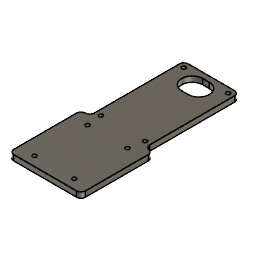
LiDAR MOUNT (Autodesk Fusion 360 design; units mm, degrees)
Autodesk Fusion 360 part; units mm, degrees
note: some values were not read from the file. Set by a fixed rule: the direction of a hole.
sketch "Sketch1" plane through (0, 0, 0) normal (0, 0, 1) x (1, 0, 0)
  line L0 (-32.5, 32.5) -> (32.5, 32.5)
  line L1 (32.5, 32.5) -> (32.5, -32.5)
  line L2 (32.5, -32.5) -> (-32.5, -32.5)
  line L3 (-32.5, -32.5) -> (-32.5, 32.5)
  point P0 (-18, 24)
  point P1 (18, 24)
  point P2 (18, -24)
  point P3 (-18, -24)
  dimension "d1" = 65
  dimension "d2" = 65
  dimension "d3" = 32.5
  dimension "d4" = 32.5
  dimension "d5" = 14.5
  dimension "d6" = 14.5
  dimension "d7" = 14.5
  dimension "d8" = 14.5
  dimension "d9" = 8.5
  dimension "d10" = 8.5
  dimension "d11" = 8.5
  dimension "d12" = 8.5
  constraint horizontal L0
  constraint vertical L1
  constraint horizontal L2
  constraint vertical L3
  measures "d1" distance of L0.start L2.end
  measures "d2" distance of L0.start L0.end
  measures "d3" distance of origin L3
  measures "d4" distance of origin L2
  measures "d5" distance of L1 P2
  measures "d6" distance of L1 P1
  measures "d7" distance of L3 P0
  measures "d8" distance of L3 P3
  measures "d9" distance of L2 P3
  measures "d10" distance of L0 P0
  measures "d11" distance of L0 P1
  measures "d12" distance of L2 P2
extrude "Extrude1" add sketch "Sketch1" along normal blind 5
hole "Hole1" at (-18, -24, 0) at (18, -24, 0) at (18, 24, 0) at (-18, 24, 0) direction (0, 0, 1) diameter 3.5 depth 5 tip angle 180 countersink diameter 6 countersink angle 90
sketch "Sketch2" plane through (0, 32.5, 0) normal (0, 1, 0) x (-1, 0, 0)
  line L0 (-32.5, 0) -> (32.5, 0)
  line L1 (32.5, 0) -> (32.5, 5)
  line L2 (32.5, 5) -> (-32.5, 5)
  line L3 (-32.5, 5) -> (-32.5, 0)
  line L4 (-25.5, 5) -> (24.5, 5)
  line L5 (24.5, 5) -> (24.5, 0)
  line L6 (24.5, 0) -> (-25.5, 0)
  line L7 (-25.5, 0) -> (-25.5, 5)
  dimension "d20" = 50
  dimension "d21" = 7
  constraint horizontal L4
  constraint vertical L5
  constraint horizontal L6
  constraint vertical L7
  constraint coincident L2 L4.start
  measures "d20" distance of L4.start L4.end
  measures "d21" distance of L3 L7
extrude "Extrude2" add sketch "Sketch2" along normal blind 85 contours L0 L2 L4 L5 L6 L7
sketch "Sketch3" plane through (0, 0, 5) normal (0, 0, 1) x (-1, 0, 0)
  circle A0 centre (-18, -24) radius 1.75
  circle A1 centre (18, 24) radius 1.75
  circle A2 centre (-18, 24) radius 1.75
  circle A3 centre (18, -24) radius 1.75
  line L0 (32.5, 32.5) -> (-32.5, 32.5)
  line L1 (-32.5, 32.5) -> (-32.5, -32.5)
  line L2 (-32.5, -32.5) -> (-25.5, -32.5)
  line L3 (-25.5, -32.5) -> (-25.5, -117.5)
  line L4 (-25.5, -117.5) -> (24.5, -117.5)
  line L5 (24.5, -117.5) -> (24.5, -32.5)
  line L6 (24.5, -32.5) -> (32.5, -32.5)
  line L7 (32.5, -32.5) -> (32.5, 32.5)
  line L8 (24.5, -32.5) -> (-25.5, -32.5) construction
  line L9 (2.5, -112.5) -> (-3.5, -112.5)
  line L10 (2.5, -93.5) -> (-3.5, -93.5)
  arc A4 (-3.5, -93.5) -> (-3.5, -112.5) centre (-3.5, -103) ccw
  arc A5 (2.5, -112.5) -> (2.5, -93.5) centre (2.5, -103) ccw
  circle A6 centre (19.5, -37.5) radius 1.75
  circle A7 centre (-20.5, -37.5) radius 1.75
  circle A8 centre (-20.5, -112.5) radius 1.75
  circle A9 centre (19.5, -112.5) radius 1.75
  point P0 (12, -103)
  point P1 (-13, -103)
  dimension "d27" = 19
  dimension "d29" = 22
  dimension "d30" = 3.5
  dimension "d31" = 3.5
  dimension "d32" = 3.5
  dimension "d33" = 3.5
  dimension "d34" = 5
  dimension "d35" = 5
  dimension "d36" = 5
  dimension "d37" = 5
  dimension "d39" = 5
  dimension "d40" = 5
  dimension "d48" = 22
  dimension "d49" = 5
  constraint coincident L5.end L6.start
  constraint coincident L2.end L3.start
  constraint tangent L9 A4
  constraint tangent L9 A5
  constraint tangent L10 A4
  constraint tangent L10 A5
  constraint horizontal A5.centre A4.centre
  constraint midpoint A5 P0
  constraint midpoint A4 P1
  measures "d27" distance of L9 L10
  measures "d29" distance of L5 A5.centre
  measures "d30" diameter of A6
  measures "d31" diameter of A7
  measures "d32" diameter of A8
  measures "d33" diameter of A9
  measures "d34" distance of L8 A6.centre
  measures "d35" distance of L5 A6.centre
  measures "d36" distance of L3 A7.centre
  measures "d37" distance of L8 A7.centre
  measures "d39" distance of L5 A9.centre
  measures "d40" distance of L3 A8.centre
  measures "d48" distance of L3 A4.centre
  measures "d49" distance of L4 L9
extrude "Extrude3" cut sketch "Sketch3" against normal blind 5 contours L9 L10 A4 A5 | A6 | A7 | A8 | A9
fillet "Fillet1" radius 4 4 edges at (25.5, 32.5, 2.5) (25.5, 117.5, 2.5) (-24.5, 117.5, 2.5) (-24.5, 32.5, 2.5)
fillet "Fillet2" radius 4 4 edges at (32.5, -32.5, 2.5) (-32.5, -32.5, 2.5) (-32.5, 32.5, 2.5) (32.5, 32.5, 2.5)
equation "d3 = ( 65 / 2 ) * 1 mm"
equation "d4 = ( 65 / 2 ) * 1 mm"
equation "d5 = 13 mm + ( 3 / 2 ) * 1 mm"
equation "d9 = 7 mm + ( ( 3 / 2 ) * 1 mm )"
equation "d21 = ( ( 64 - 50 ) / 2 ) * 1 mm"
equation "d27 = 23.5 mm - 4.5 mm"
